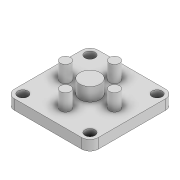
# Autodesk Inventor part: PDMS stretcher mould A (x4)
Saved by Autodesk Inventor 2020 (Build 240168000, 168)
## iProperties
Created: 2022-05-16
Part Number: PDMS stretcher mould A (x4)
Material: Generic
Document SubType Name: Modeling
Designer: ferrerx
Density: 1 g/cm^3
Appearance: Default
Author: ferrerx
Autodesk Inventor part; units mm, degrees
ref_plane "YZ Plane" through (0, 0, 0) normal (1, 0, 0) x (0, 1, 0)
ref_plane "XZ Plane" through (0, 0, 0) normal (0, 1, 0) x (-1, 0, 0)
ref_plane "XY Plane" through (0, 0, 0) normal (0, 0, 1) x (1, 0, 0)
sketch "Sketch1" plane through (0, 0, 0) normal (0, 1, 0) x (-1, 0, 0)
  line L0 (-12.5, 12.5) -> (12.5, 12.5)
  line L1 (12.5, 12.5) -> (12.5, -12.5)
  line L2 (12.5, -12.5) -> (-12.5, -12.5)
  line L3 (-12.5, -12.5) -> (-12.5, 12.5)
  line L4 (-12.5, 12.5) -> (12.5, -12.5) construction
  line L5 (12.5, 12.5) -> (-12.5, -12.5) construction
  line L6 (-10, 10) -> (10, 10) construction
  line L7 (10, 10) -> (10, -10) construction
  line L8 (10, -10) -> (-10, -10) construction
  line L9 (-10, -10) -> (-10, 10) construction
  line L10 (-10, 10) -> (10, -10) construction
  line L11 (10, 10) -> (-10, -10) construction
  circle A0 centre (10, 10) radius 1.5
  circle A1 centre (10, -10) radius 1.5
  circle A2 centre (-10, -10) radius 1.5
  circle A3 centre (-10, 10) radius 1.5
  point P0 (0, 0)
  dimension "d0" = 25
  dimension "d1" = 25
  dimension "d2" = 3
  dimension "d3" = 3
  dimension "d4" = 3
  dimension "d5" = 3
  dimension "d6" = 20
  constraints: 24 end point, 4 centre point, 4 coincident, 4 midpoint, 4 parallel, 2 horizontal, 2 perpendicular, 1 point on line
  measures "d0" distance of L1.end L2.end
  measures "d1" distance of L0.end L1.end
  measures "d2" diameter of A0
  measures "d3" diameter of A1
  measures "d4" diameter of A3
  measures "d5" diameter of A2
  measures "d6" distance of L7.end L8.end
extrude "Extrusion1" add sketch "Sketch1" along normal blind 3
sketch "Sketch2" plane through (0, 3, 0) normal (0, 1, 0) x (1, 0, 0)
  circle A0 centre (0, 0) radius 3
  circle A1 centre (-5.5, 0) radius 1.5
  circle A2 centre (-2.75, -4.7631) radius 1.5
  circle A3 centre (2.75, -4.7631) radius 1.5
  circle A4 centre (5.5, 0) radius 1.5
  circle A5 centre (2.75, 4.7631) radius 1.5
  circle A6 centre (-2.75, 4.7631) radius 1.5
  dimension "d9" = 6
  dimension "d10" = 3
  dimension "d11" = 5.5
  dimension "d14" = 360
  constraints: 7 centre point, 1 coincident, 13 other
  measures "d9" diameter of A0
  measures "d10" diameter of A1
  measures "d11" distance of A0.centre A1.centre
extrude "Extrusion2" add sketch "Sketch2" along normal blind 5 contours A1 | A2 | A3 | A4 | A5 | A6
sketch "Sketch3" plane through (0, 3, 0) normal (0, 1, 0) x (1, 0, 0)
  circle A0 centre (0, 0) radius 3
  dimension "d18" = 6
  constraints: 1 centre point, 1 coincident
  measures "d18" diameter of A0
extrude "Extrusion3" add sketch "Sketch3" along normal blind 4
sketch "Sketch5" plane through (-5.5, 8, 0) normal (0, 1, 0) x (1, 0, 0)
  circle A0 centre (0, 0) radius 2.5
  circle A1 centre (2.75, -4.7631) radius 2.5
  circle A2 centre (8.25, -4.7631) radius 2.5
  circle A3 centre (11, 0) radius 2.5
  circle A4 centre (8.25, 4.7631) radius 2.5
  circle A5 centre (2.75, 4.7631) radius 2.5
  circle A6 centre (5.5, 0) radius 3.5
  circle A7 centre (0, 0) radius 1.4875
  circle A8 centre (2.75, -4.7631) radius 1.4875
  circle A9 centre (8.25, -4.7631) radius 1.4875
  circle A10 centre (11, 0) radius 1.4875
  circle A11 centre (8.25, 4.7631) radius 1.4875
  circle A12 centre (2.75, 4.7631) radius 1.4875
  line L0 (18, 12.5) -> (-7, 12.5) projected
  line L1 (18, -12.5) -> (-7, -12.5)
  line L2 (-7, -12.5) -> (-7, 12.5)
  line L3 (-7, 12.5) -> (18, 12.5)
  line L4 (18, 12.5) -> (18, -12.5)
  line L5 (18, -12.5) -> (-7, 12.5) construction
  line L6 (-7, -12.5) -> (18, 12.5) construction
  circle A13 centre (-4.5, -10) radius 1.5 projected
  circle A14 centre (-4.5, -10) radius 1.65
  circle A15 centre (-4.5, 10) radius 1.5 projected
  circle A16 centre (-4.5, 10) radius 1.65
  circle A17 centre (15.5, 10) radius 1.5 projected
  circle A18 centre (15.5, 10) radius 1.65
  circle A19 centre (15.5, -10) radius 1.5 projected
  circle A20 centre (15.5, -10) radius 1.65
  point P0 (8.7955, -1.179)
  point P1 (8.1687, -2.2645)
  point P2 (6.1267, -3.4434)
  point P3 (4.8733, -3.4434)
  point P4 (2.8313, -2.2645)
  point P5 (2.2045, -1.179)
  point P6 (2.2045, 1.179)
  point P7 (2.8313, 2.2645)
  point P8 (4.8733, 3.4434)
  point P9 (6.1267, 3.4434)
  point P10 (8.1687, 2.2645)
  point P11 (8.7955, 1.179)
  dimension "d21" = 5
  dimension "d24" = 360
  dimension "d26" = 7
  dimension "d29" = 360
  constraints: 17 centre point, 12 end point, 6 coincident, 2 midpoint, 2 parallel, 1 horizontal, 1 perpendicular, 26 other
  measures "d21" diameter of A0
  measures "d26" diameter of A6
extrude "Extrusion4" add sketch "Sketch5" against normal blind 5 contours L4 L1 L2 L0 | A14 | A16 | A18 | A20
fillet "Fillet1" radius 0.5 12 edges at (-2.6687, 5.5, 2.2645) (-0.6267, 5.5, 3.4434) (2.6687, 5.5, 2.2645) (0.6267, 5.5, 3.4434) (-3.2955, 5.5, -1.179) (-3.2955, 5.5, 1.179) (-0.6267, 5.5, -3.4434) (-2.6687, 5.5, -2.2645) (2.6687, 5.5, -2.2645) (0.6267, 5.5, -3.4434) (3.2955, 5.5, 1.179) (3.2955, 5.5, -1.179)
fillet "Fillet2" radius 2.5 4 edges at (12.5, 4, -12.5) (-12.5, 4, -12.5) (12.5, 4, 12.5) (-12.5, 4, 12.5)
sketch "Sketch7" plane through (0, 7, 0) normal (0, 1, 0) x (1, 0, 0)
  circle A0 centre (0, 0) radius 1
  constraints: 1 centre point, 1 coincident
extrude "Extrusion5" [suppressed]
sketch "Sketch8" plane through (-5.5, 8, 0) normal (0, 1, 0) x (1, 0, 0)
  circle A0 centre (0, 0) radius 1
  point P0 (5.5, 0)
  dimension "d37" = 2
  constraints: 1 centre point
  measures "d37" diameter of A0
extrude "Extrusion6" [suppressed]
pattern_circular "Circular Pattern1" [suppressed]
sketch "Sketch9" plane through (-5.5, 8, 0) normal (0, 1, 0) x (1, 0, 0)
  line L0 (-7.0276, -1) -> (-2, -1)
  line L1 (-2, -1) -> (-2, 1)
  line L2 (-2, 1) -> (-7.0276, 1)
  line L3 (-7.0276, 1) -> (-7.0276, -1)
  line L4 (-7.0276, -1) -> (-2, 1) construction
  line L5 (-2, -1) -> (-7.0276, 1) construction
  point P0 (5.5, 0)
  point P1 (-4.5138, 0)
  constraints: 12 end point, 2 midpoint, 2 parallel, 1 horizontal, 1 perpendicular
extrude "Extrusion7" cut sketch "Sketch9" against normal blind 5
thicken "Thicken1" operation add thickness 5 both sides no extend neighbours yes toward (0, -1, 0) faces at (0.7594, 8, 10.7394)
sketch "Sketch10" plane through (5.5, 8, 0) normal (0, 1, 0) x (1, 0, 0)
  circle A0 centre (-5.5, 0) radius 3.2016
  circle A1 centre (-5.5, 0) radius 8.2006
  constraints: 2 centre point, 2 coincident
extrude "Extrusion8" cut sketch "Sketch10" against normal blind 5
sketch "Sketch12" plane through (-10, 3, 12.5) normal (0, 1, 0) x (1, 0, 0)
  circle A0 centre (10, 12.5) radius 7.3 construction
  circle A1 centre (10, 19.8) radius 1.5
  dimension "d49" = 14.6
  dimension "d50" = 3
  constraints: 1 centre point, 1 coincident, 1 vertical alignment, 2 other
  measures "d50" diameter of A1
extrude "Extrusion9" add sketch "Sketch12" along normal blind 5
pattern_circular "Circular Pattern2" count 4 over 360 about axis through (0, 3, 0) along (0, 1, 0) of "Extrusion9"
body "Solid1"
